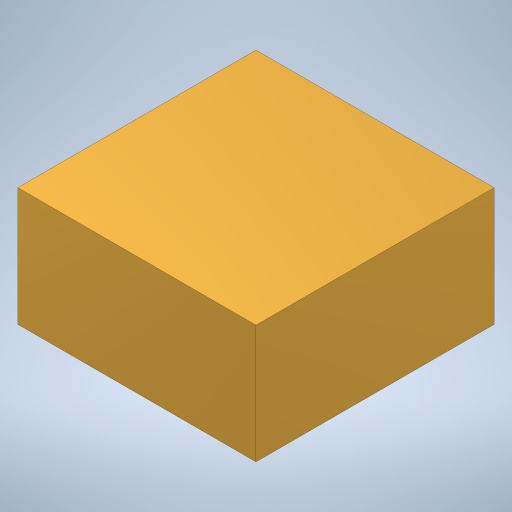
# Autodesk Inventor part: cube
Saved by Autodesk Inventor 2023 (Build 270158000, 158)
## iProperties
Created: 2022-06-16
Part Number: cube
Material: Brass, Soft Yellow
Document SubType Name: Modeling
Designer: TRIVENI MAGADUM
Density: 8.47 g/cm^3
Appearance: Brass - Satin
Author: TRIVENI MAGADUM
Autodesk Inventor part; units mm, degrees
ref_plane "YZ Plane" through (0, 0, 0) normal (1, 0, 0) x (0, 1, 0)
ref_plane "XZ Plane" through (0, 0, 0) normal (0, 1, 0) x (-1, 0, 0)
ref_plane "XY Plane" through (0, 0, 0) normal (0, 0, 1) x (1, 0, 0)
sketch "Sketch1" plane through (0, 0, 0) normal (0, 1, 0) x (-1, 0, 0)
  point P0 (0, 0)
sketch "Sketch2" plane through (0, 0, 0) normal (0, 1, 0) x (-1, 0, 0)
  point P0 (0, 0)
sketch "Sketch3" plane through (0, 0, 0) normal (0, 1, 0) x (-1, 0, 0)
  line L0 (4.7625, 4.7625) -> (-35.2375, 4.7625)
  line L1 (-35.2375, 4.7625) -> (-35.2375, -35.2375)
  line L2 (-35.2375, -35.2375) -> (4.7625, -35.2375)
  line L3 (4.7625, -35.2375) -> (4.7625, 4.7625)
  point P0 (0, 0)
  dimension "d0" = 40
  dimension "d1" = 40
  constraints: 8 end point, 2 parallel, 1 horizontal, 1 perpendicular
  measures "d0" distance of L2.end L1.end
  measures "d1" distance of L1.end L0.end
extrude "Extrusion1" add sketch "Sketch3" along normal blind 19.885
body "Solid1"
